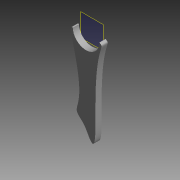
# Autodesk Inventor part: body02
Saved by Autodesk Inventor 2013 (Build 170138000, 138)
## iProperties
Created: 2013-02-19
Part Number: body02
Material: Generic
Document SubType Name: Modeling
Designer: Nano
Density: 1 g/cm^3
Author: Nano
Autodesk Inventor part; units mm, degrees
ref_plane "YZ Plane" through (0, 0, 0) normal (1, 0, 0) x (0, 1, 0)
ref_plane "XZ Plane" through (0, 0, 0) normal (0, 1, 0) x (-1, 0, 0)
ref_plane "XY Plane" through (0, 0, 0) normal (0, 0, 1) x (1, 0, 0)
ref_plane "Work Plane1" through (0, 0, -22.225) normal (0, 0, -1) x (-1, 0, 0)
sketch "Sketch1" plane through (0, 0, -22.225) normal (0, 0, -1) x (-1, 0, 0)
  circle A0 centre (0, 0) radius 150.593
  spline S0 degree 4 poles (150.5264, -4.4762) (213.9602, 25.4861) (80.5156, -314.2865) (42.4775, -681.7659) (139.8238, -807.3182) (20.435, -872.5986) (-25.019, -981.8143) (-175.111, -1238.1839) (-34.5572, -17.9805) (-234.4483, -34.8604) (-150.593, 0) knots 0 0 0 0 0 0.241647 0.346741 0.430496 0.500884 0.602185 0.725781 1 1 1 1 1
  point P0 (170.3977, -23.7077)
  point P1 (83.4122, -476.7037)
  point P2 (99.1023, -747.7959)
  point P3 (99.1025, -812.4322)
  point P4 (43.0812, -871.0509)
  point P5 (-17.4153, -958.4347)
  point P6 (-70.261, -1031.201)
  point P7 (-111.5208, -446.1599)
  point P8 (-175.9798, -23.7077)
  constraints: 2 point on circle, 1 centre point, 1 coincident, 11 other
extrude "Extrusion1" add sketch "Sketch1" against normal blind 69.85 contours A0 S0
body "Solid1"
